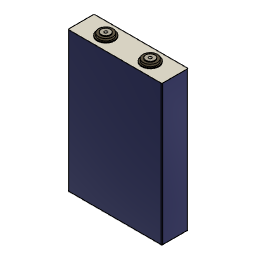
105Ah LiFePO4 cell (Autodesk Fusion 360 design; units mm, degrees)
Autodesk Fusion 360 part; units mm, degrees
note: some values were not read from the file. Set by a fixed rule: which sketch regions a step uses.
sketch "Sketch1" plane through (0, 0, 0) normal (0, 0, 1) x (1, 0, 0)
  line L0 (0, 0) -> (131, 0)
  line L1 (131, 0) -> (131, 36.5)
  line L2 (131, 36.5) -> (0, 36.5)
  line L3 (0, 36.5) -> (0, 0)
  line L4 (65.5, 18.25) -> (96.5, 18.25)
  line L5 (65.5, 18.25) -> (34.5, 18.25)
  circle A0 centre (34.5, 18.25) radius 12
  circle A1 centre (96.5, 18.25) radius 12
  circle A2 centre (34.5, 18.25) radius 10
  circle A3 centre (96.5, 18.25) radius 10
  circle A4 centre (34.5, 18.25) radius 6.5
  circle A5 centre (96.5, 18.25) radius 6.5
  circle A6 centre (34.5, 18.25) radius 2
  circle A7 centre (96.5, 18.25) radius 2
  dimension "d1" = 131
  dimension "d2" = 36.5
  dimension "d3" = 31
  dimension "d4" = 31
  dimension "d5" = 24
  dimension "d6" = 24
  dimension "d7" = 20
  dimension "d8" = 20
  dimension "d9" = 13
  dimension "d10" = 13
  dimension "d17" = 4
  dimension "d18" = 4
  constraint horizontal L0
  constraint vertical L1
  constraint horizontal L2
  constraint vertical L3
  constraint coincident L0.start L3.end
  constraint perpendicular L3 L4
  constraint parallel L4 L5
  constraint coincident L5.end A0.centre
  constraint coincident L4.end A1.centre
  constraint concentric A0 A2
  constraint concentric A1 A3
  constraint concentric A0 A4
  constraint concentric A3 A5
  constraint concentric A2 A6
  constraint concentric A3 A7
  measures "d1" distance of L0.start L0.end
  measures "d2" distance of L0.start L2.end
  measures "d3" distance of L4.start L4.end
  measures "d4" distance of L4.start L5.end
  measures "d5" diameter of A0
  measures "d6" diameter of A1
  measures "d7" diameter of A2
  measures "d8" diameter of A3
  measures "d9" diameter of A4
  measures "d10" diameter of A5
  measures "d17" diameter of A6
  measures "d18" diameter of A7
extrude "Extrude1" add sketch "Sketch1" against normal blind 196 contours L0 L1 L2 L3 | A0 | A1 | A2 | A3 | A4 | A5 | A6 | A7
extrude "Extrude2" add sketch "Sketch1" along normal blind 1 contours A0 | A1
extrude "Extrude3" add sketch "Sketch1" along normal blind 4 contours A2 | A3
extrude "Extrude4" add sketch "Sketch1" along normal blind 5 contours A4 | A5
fillet "Fillet1" radius 1 4 edges at (0, 0, -98) (131, 0, -98) (131, 36.5, -98) (0, 36.5, -98) 1 faces at (43.6667, 12.1667, -196)
equation "d3 = ( 62 / 2 ) * 1 mm"
equation "d4 = ( 62 / 2 ) * 1 mm"
